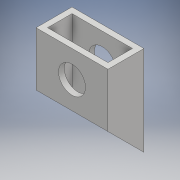
# Autodesk Inventor part: Pipe4
Saved by Autodesk Inventor 2018 (Build 220112000, 112)
## iProperties
Created: 2017-09-10
Part Number: Pipe4
Material: 一般
Document SubType Name: Modeling
Designer: mura5
Density: 1 g/cm^3
Appearance: 既定
Author: mura5
Autodesk Inventor part; units mm, degrees
ref_plane "YZ Plane" through (0, 0, 0) normal (1, 0, 0) x (0, 1, 0)
ref_plane "XZ Plane" through (0, 0, 0) normal (0, 1, 0) x (-1, 0, 0)
ref_plane "XY Plane" through (0, 0, 0) normal (0, 0, 1) x (1, 0, 0)
sketch "スケッチ1" plane through (0, 0, 0) normal (0, 0, 1) x (1, 0, 0)
  line L0 (-20, -10) -> (20, -10)
  line L1 (20, -10) -> (20, 10)
  line L2 (20, 10) -> (-20, 10)
  line L3 (-20, 10) -> (-20, -10)
  line L4 (-20, -10) -> (20, 10) construction
  line L5 (20, -10) -> (-20, 10) construction
  line L6 (-16.8, 6.8) -> (16.8, 6.8)
  line L7 (16.8, 6.8) -> (16.8, -6.8)
  line L8 (16.8, -6.8) -> (-16.8, -6.8)
  line L9 (-16.8, -6.8) -> (-16.8, 6.8)
  point P0 (0, 0)
  dimension "d0" = 40
  dimension "d1" = 20
  dimension "d2" = 3.2
  constraints: 20 end point, 4 parallel, 2 midpoint, 2 perpendicular, 1 horizontal, 3 other
  measures "d0" distance of L2.end L1.end
  measures "d1" distance of L1.end L0.end
  measures "d2" distance between parallel lines of L2 L6
extrude "押し出し1" add sketch "スケッチ1" along normal blind 50
chamfer "面取り1" distance 20 angle 45 1 edges at (0, -10, 0)
sketch "スケッチ2" plane through (-20, -10, 50) normal (0, -1, 0) x (1, 0, 0)
  line L0 (0, 0) -> (40, 0) projected
  line L1 (40, -30) -> (40, 0) projected
  point P0 (20, -50)
  point P1 (20, -15)
  dimension "d9" = 15
  dimension "d10" = 20
  measures "d9" distance from line of L0 point (20, -15)
  measures "d10" distance from line of L1 point (20, -15)
hole "穴1" at (0, -10, 35) direction (0, 1, 0) diameter 15 end through all
